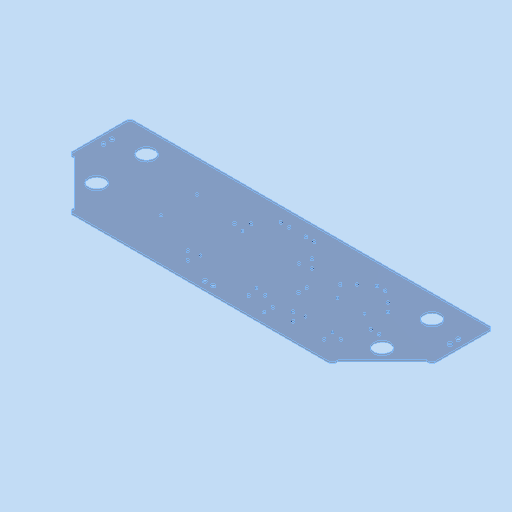
# Autodesk Inventor part: enc-ElectronicsPanel V1
Saved by Autodesk Inventor 2023.2 (Build 272271000, 271)
## iProperties
Created: 2023-11-30
Part Number: enc-ElectronicsPanel V1
Material: Generisch
Document SubType Name: Modeling
Designer: Nils Bade
Density: 1 g/cm^3
Appearance: PVC Verglasung
Description: Fertigung
Auf Bestellliste: True
Author: Nils Bade
Autodesk Inventor part; units mm, degrees
ref_plane "YZ Plane" through (0, 0, 0) normal (1, 0, 0) x (0, 1, 0)
ref_plane "XZ Plane" through (0, 0, 0) normal (0, 1, 0) x (-1, 0, 0)
ref_plane "XY Plane" through (0, 0, 0) normal (0, 0, 1) x (1, 0, 0)
sketch "Skizze1" plane through (0, 0, 0) normal (0, 1, 0) x (-1, 0, 0)
  line L0 (0, 0) -> (-655, 0)
  line L1 (-655, 0) -> (-655, 200)
  line L2 (-655, 200) -> (0, 200)
  line L3 (0, 200) -> (0, 0)
  line L4 (-327.5, 0) -> (-327.5, 200) construction
  line L5 (0, 100) -> (-655, 100) construction
  line L6 (-655, 55) -> (0, 55) construction
  line L7 (0, 80) -> (-655, 80) construction
  line L8 (-640, 185) -> (-640, 15) construction
  line L9 (-640, 15) -> (-15, 15) construction
  line L10 (-15, 15) -> (-15, 185) construction
  line L11 (-15, 185) -> (-640, 185) construction
  circle A0 centre (-15, 47.5) radius 3.25
  circle A1 centre (-15, 62.5) radius 3.25
  circle A2 centre (-320, 185) radius 3.25
  circle A3 centre (-335, 185) radius 3.25
  circle A4 centre (-640, 47.5) radius 3.25
  circle A5 centre (-640, 62.5) radius 3.25
  line L12 (-90, 200) -> (-90, 190)
  line L13 (-90, 190) -> (-10, 110)
  line L14 (-10, 110) -> (0, 110)
  line L15 (-565, 200) -> (-565, 190)
  line L16 (-565, 190) -> (-645, 110)
  line L17 (-645, 110) -> (-655, 110)
  circle A6 centre (-70, 130) radius 15
  circle A7 centre (-70, 40) radius 15
  circle A8 centre (-585, 130) radius 15
  circle A9 centre (-585, 40) radius 15
  point P0 (-15, 55)
  point P1 (-327.5, 185)
  point P2 (-565, 200)
  point P3 (-655, 110)
  dimension "d0" = 655
  dimension "d1" = 200
  dimension "d2" = 145
  dimension "d3" = 80
  dimension "d6" = 15
  dimension "d13" = 6.5
  dimension "d14" = 7.5
  dimension "d21" = 6.5
  dimension "d23" = 7.5
  dimension "d80" = 625
  dimension "d81" = 45
  dimension "d83" = 90
  dimension "d84" = 90
  dimension "d85" = 10
  dimension "d86" = 30
  dimension "d87" = 70
  dimension "d88" = 70
  dimension "d91" = 90
  constraints: 36 end point, 10 centre point, 10 point on line, 10 symmetric about line, 5 midpoint, 5 perpendicular, 4 parallel, 2 vertical, 1 horizontal, 11 other
  measures "d0" distance of L0.start L0.end
  measures "d1" distance of L2.end L0.start
  measures "d2" distance between parallel lines of L2 L6
  measures "d3" distance between parallel lines of L0 L7
  measures "d6" distance between parallel lines of L1 L8
  measures "d13" diameter of A0
  measures "d14" distance from line of L6 A0.centre
  measures "d21" diameter of A2
  measures "d23" distance from line of L4 A2.centre
  measures "d80" distance between parallel lines of L8 L10
  measures "d81" angle of L2 L13
  measures "d83" distance between parallel lines of L3 L12
  measures "d84" distance between parallel lines of L2 L14
  measures "d85" distance of L12.start L12.end
  measures "d86" diameter of A6
  measures "d87" distance from line of A6.centre L2
  measures "d88" distance from line of L3 A6.centre
  measures "d91" distance of A6.centre A7.centre
extrude "Ex-Platte" add sketch "Skizze1" along normal blind 3 contours L0 L1 L17 L16 L15 L2 L12 L13 L14 L3
sketch "S-Anschraubpunkte" plane through (0, 0, 0) normal (0, 1, 0) x (-1, 0, 0)
  line L0 (-655, 0) -> (0, 0) construction
  line L1 (-90, 200) -> (-565, 200) construction
  line L2 (-655, 0) -> (0, 0) construction
  line L3 (-327.5, 0) -> (-327.5, 200) construction
  line L4 (-129.8577, 12.8998) -> (-226.8577, 12.8998) construction
  line L5 (-226.8577, 12.8998) -> (-226.8577, 171.8998) construction
  line L6 (-226.8577, 171.8998) -> (-129.8577, 171.8998) construction
  line L7 (-129.8577, 171.8998) -> (-129.8577, 12.8998) construction
  line L8 (-272.665, 68.869) -> (-382.335, 68.869) construction
  line L9 (-382.335, 68.869) -> (-382.335, 153.169) construction
  line L10 (-382.335, 153.169) -> (-272.665, 153.169) construction
  line L11 (-272.665, 153.169) -> (-272.665, 68.869) construction
  line L12 (-463.0213, 68.519) -> (-519.0213, 68.519) construction
  line L13 (-519.0213, 68.519) -> (-519.0213, 153.519) construction
  line L14 (-519.0213, 153.519) -> (-463.0213, 153.519) construction
  line L15 (-463.0213, 153.519) -> (-463.0213, 68.519) construction
  line L16 (-491.0213, 68.519) -> (-491.0213, 153.519) construction
  line L17 (-463.0213, 111.019) -> (-519.0213, 111.019) construction
  line L18 (-327.5, 68.869) -> (-327.5, 153.169) construction
  line L19 (-272.665, 111.019) -> (-382.335, 111.019) construction
  line L20 (-178.3577, 12.8998) -> (-178.3577, 171.8998) construction
  line L21 (-226.8577, 92.3998) -> (-129.8577, 92.3998) construction
  circle A0 centre (-466.5213, 150.019) radius 1.35
  circle A1 centre (-448.0213, 68.519) radius 2.15
  circle A2 centre (-463.0213, 53.519) radius 2.15
  circle A3 centre (-534.0213, 68.519) radius 2.15
  circle A4 centre (-519.0213, 53.519) radius 2.15
  circle A5 centre (-448.0213, 153.519) radius 2.15
  circle A6 centre (-463.0213, 168.519) radius 2.15
  circle A7 centre (-519.0213, 168.519) radius 2.15
  circle A8 centre (-534.0213, 153.519) radius 2.15
  circle A9 centre (-276.645, 149.169) radius 1.65
  circle A10 centre (-276.645, 73.069) radius 1.65
  circle A11 centre (-377.995, 73.069) radius 1.65
  circle A12 centre (-377.995, 149.169) radius 1.65
  circle A13 centre (-257.665, 153.169) radius 2.15
  circle A14 centre (-272.665, 168.169) radius 2.15
  circle A15 centre (-257.665, 68.869) radius 2.15
  circle A16 centre (-272.665, 53.869) radius 2.15
  circle A17 centre (-397.335, 153.169) radius 2.15
  circle A18 centre (-382.335, 168.169) radius 2.15
  circle A19 centre (-382.335, 53.869) radius 2.15
  circle A20 centre (-397.335, 68.869) radius 2.15
  circle A21 centre (-178.3577, 122.1498) radius 1.65
  circle A22 centre (-178.3577, 57.1498) radius 1.65
  circle A23 centre (-515.5213, 150.019) radius 1.35
  circle A24 centre (-466.5213, 92.019) radius 1.35
  circle A25 centre (-515.5213, 92.019) radius 1.35
  circle A26 centre (-422.6782, 165) radius 2.15
  circle A27 centre (-422.6782, 180) radius 2.15
  line L22 (-422.6782, 165) -> (-422.6782, 180) construction
  circle A28 centre (-560.7476, 111.019) radius 2.15
  circle A29 centre (-545.7476, 111.019) radius 2.15
  line L23 (-560.7476, 111.019) -> (-545.7476, 111.019) construction
  circle A30 centre (-297.5, 25.1204) radius 2.15
  circle A31 centre (-312.5, 25.1204) radius 2.15
  line L24 (-297.5, 25.1204) -> (-312.5, 25.1204) construction
  circle A32 centre (-342.5, 25.1204) radius 2.15
  circle A33 centre (-357.5, 25.1204) radius 2.15
  line L25 (-342.5, 25.1204) -> (-357.5, 25.1204) construction
  circle A34 centre (-498.5213, 37.836) radius 2.15
  circle A35 centre (-483.5213, 37.836) radius 2.15
  line L26 (-498.5213, 37.836) -> (-483.5213, 37.836) construction
  circle A36 centre (-422.6782, 103.519) radius 2.15
  circle A37 centre (-422.6782, 118.519) radius 2.15
  line L27 (-422.6782, 103.519) -> (-422.6782, 118.519) construction
  line L28 (-312.5, 25.1204) -> (-342.5, 25.1204) construction
  point P0 (-422.6782, 111.019)
  point P1 (-491.0213, 37.836)
  point P2 (-327.5, 25.1204)
  dimension "d96" = 97
  dimension "d97" = 159
  dimension "d98" = 109.67
  dimension "d99" = 84.3
  dimension "d100" = 56
  dimension "d101" = 85
  dimension "d102" = 2.7
  dimension "d105" = 4.3
  dimension "d106" = 4.3
  dimension "d107" = 15
  dimension "d108" = 15
  dimension "d110" = 3.98
  dimension "d111" = 3.3
  dimension "d112" = 4
  dimension "d115" = 76.1
  dimension "d122" = 101.35
  dimension "d127" = 4.3
  dimension "d128" = 4.3
  dimension "d129" = 15
  dimension "d130" = 15
  dimension "d132" = 49.75
  dimension "d135" = 65
  dimension "d140" = 3.3
  dimension "d154" = 3.5
  dimension "d155" = 3.5
  dimension "d158" = 58
  dimension "d174" = 4.3
  dimension "d176" = 4.3
  dimension "d177" = 15
  dimension "d178" = 20
  dimension "d195" = 4.3
  dimension "d196" = 4.3
  dimension "d197" = 15
  dimension "d214" = 4.3
  dimension "d215" = 4.3
  dimension "d216" = 15
  dimension "d233" = 4.3
  dimension "d234" = 4.3
  dimension "d235" = 15
  dimension "d252" = 4.3
  dimension "d253" = 4.3
  dimension "d254" = 15
  dimension "d271" = 4.3
  dimension "d272" = 4.3
  dimension "d273" = 15
  dimension "d274" = 30
  constraints: 52 end point, 38 centre point, 17 midpoint, 13 symmetric about line, 9 horizontal, 8 point on line, 6 parallel, 5 collinear, 5 vertical, 3 perpendicular, 26 other
  measures "d96" distance between parallel lines of L7 L5
  measures "d97" distance between parallel lines of L6 L4
  measures "d98" distance of L8.start L8.end
  measures "d99" distance of L10.end L8.start
  measures "d100" distance of L12.start L12.end
  measures "d101" distance of L12.end L13.end
  measures "d102" diameter of A0
  measures "d105" diameter of A1
  measures "d106" diameter of A2
  measures "d107" distance from line of L12 A2.centre
  measures "d108" distance from line of L15 A1.centre
  measures "d110" distance from line of L11 A9.centre
  measures "d111" diameter of A9
  measures "d112" distance from line of L10 A9.centre
  measures "d115" distance of A9.centre A10.centre
  measures "d122" distance of A10.centre A11.centre
  measures "d127" diameter of A13
  measures "d128" diameter of A14
  measures "d129" distance from line of L10 A14.centre
  measures "d130" distance from line of L11 A13.centre
  measures "d132" distance from line of L6 A21.centre
  measures "d135" distance of A21.centre A22.centre
  measures "d140" diameter of A21
  measures "d154" distance from line of L15 A0.centre
  measures "d155" distance from line of L14 A0.centre
  measures "d158" distance of A0.centre A24.centre
  measures "d174" diameter of A26
  measures "d176" diameter of A27
  measures "d177" distance of L22.end L22.start
  measures "d178" distance from line of L1 L22.end
  measures "d195" diameter of A28
  measures "d196" diameter of A29
  measures "d197" distance of L23.end L23.start
  measures "d214" diameter of A30
  measures "d215" diameter of A31
  measures "d216" distance of L24.end L24.start
  measures "d233" diameter of A32
  measures "d234" diameter of A33
  measures "d235" distance of L25.end L25.start
  measures "d252" diameter of A34
  measures "d253" diameter of A35
  measures "d254" distance of L26.end L26.start
  measures "d271" diameter of A36
  measures "d272" diameter of A37
  measures "d273" distance of L27.end L27.start
  measures "d274" distance of L24.end L25.start
extrude "Ex-Anschraubpunkte" cut sketch "S-Anschraubpunkte" along normal blind 3
chamfer "Fase-5mm" distance 5 angle 45 6 edges at (655, 1.5, 0) (0, 1.5, 0) (0, 1.5, 110) (90, 1.5, 200) (565, 1.5, 200) (655, 1.5, 110)
equation "\"d21\" = d13"
equation "\"d23\" = d14"
equation "\"d84\" = d83"
